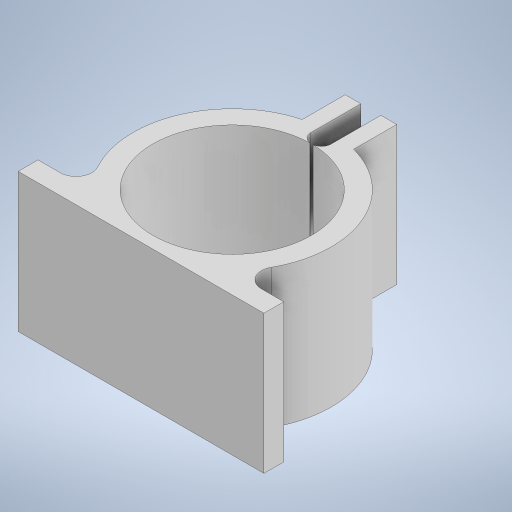
# Autodesk Inventor part: MotorClamp
Saved by Autodesk Inventor 2024 (Build 280153000, 153)
## iProperties
Created: 2023-08-28
Part Number: MotorClamp
Material: Generic
Document SubType Name: Modeling
Designer: KirikDK
Density: 1 g/cm^3
Appearance: Default
Author: KirikDK
Autodesk Inventor part; units mm, degrees
ref_plane "YZ Plane" through (0, 0, 0) normal (1, 0, 0) x (0, 1, 0)
ref_plane "XZ Plane" through (0, 0, 0) normal (0, 1, 0) x (-1, 0, 0)
ref_plane "XY Plane" through (0, 0, 0) normal (0, 0, 1) x (1, 0, 0)
sketch "Sketch1" plane through (0, 0, 0) normal (0, 1, 0) x (-1, 0, 0)
  circle A0 centre (0, 0) radius 50
  circle A1 centre (0, 0) radius 40
  line L0 (50, 0) -> (-50, 0)
  line L1 (-50, 0) -> (-50, 50)
  line L2 (-50, 50) -> (50, 50)
  line L3 (50, 50) -> (50, 0)
  line L4 (6, -46) -> (-6, -46)
  line L5 (-6, -46) -> (-6, -62)
  line L6 (-6, -62) -> (6, -62)
  line L7 (6, -62) -> (6, -46)
  line L8 (1, -64) -> (-1, -64)
  line L9 (-1, -64) -> (-1, -35)
  line L10 (-1, -35) -> (1, -35)
  line L11 (1, -35) -> (1, -64)
  point P0 (1, -39.9875)
  point P1 (1, -62)
  point P2 (6, -49.6387)
  point P3 (-6, -49.6387)
  point P4 (-1, -62)
  point P5 (-1, -39.9875)
  dimension "d0" = 100
  constraints: 24 end point, 6 parallel, 3 horizontal, 3 perpendicular, 2 coincident, 1 centre point, 3 other
extrude "Extrusion1" add sketch "Sketch1" along normal blind 70 contours L0 A1 A0 | A0 L7 L4 L11 A1 L0 | A0 L2 L3 | A0 L1 L2 | L7 L6 L11 A0 | A0 L11 L4 L7 | L0 A1 L9 L4 L5 A0 | L5 L4 L9 A0 | A0 L9 L6 L5
sketch "Sketch2" plane through (0, 70, 0) normal (0, 1, 0) x (1, 0, 0)
  circle A0 centre (0, 62) radius 3.05
  dimension "d9" = 6.1
  constraints: 1 centre point
  measures "d9" diameter of A0
extrude "Extrusion2" cut sketch "Sketch2" against normal blind 100
sketch "Sketch3" plane through (0, 70, 0) normal (0, 1, 0) x (1, 0, 0)
  line L0 (-3.05, 48) -> (-8, 48)
  line L1 (-8, 48) -> (-8, 62.2274)
  line L2 (-8, 62.2274) -> (-3.05, 62.2274)
  line L3 (-3.05, 62.2274) -> (-3.05, 48)
  line L4 (3.0501, 48) -> (8, 48)
  line L5 (8, 48) -> (8, 62.2274)
  line L6 (8, 62.2274) -> (3.0501, 62.2274)
  line L7 (3.0501, 62.2274) -> (3.0501, 48)
  constraints: 16 end point, 4 parallel, 2 horizontal, 2 perpendicular, 2 point on line
extrude "Extrusion3" add sketch "Sketch3" against normal up to surface (70 mm away)
sketch "Sketch4" plane through (0, 70, 0) normal (0, 1, 0) x (1, 0, 0)
  line L0 (8, 62.2274) -> (3.0501, 62.2274) construction
  line L1 (-3.05, 62.2274) -> (-8, 62.2274) construction
  arc A0 (-8, 49.3559) -> (-50, 0) centre (0, 0) ccw construction
  arc A1 (50, 0) -> (8, 49.3559) centre (0, 0) ccw construction
  line L2 (-8, 62.2274) -> (-20.0044, 45.8238)
  line L3 (8, 62.2274) -> (20.0044, 45.8238)
  line L4 (-20.0044, 45.8238) -> (-5.525, 45.8238)
  line L5 (-5.525, 45.8238) -> (-5.525, 62.2274)
  line L6 (-8, 62.2274) -> (-5.525, 62.2274)
  line L7 (20.0044, 45.8238) -> (5.5251, 45.8238)
  line L8 (5.5251, 45.8238) -> (5.5251, 62.2274)
  line L9 (5.5251, 62.2274) -> (8, 62.2274)
  constraints: 16 end point, 2 midpoint, 2 point on circle, 1 collinear, 1 horizontal, 1 perpendicular, 1 point on line
extrude "Extrusion4" add sketch "Sketch4" against normal blind 6
sketch "Sketch6" plane through (0, 70, 0) normal (0, 1, 0) x (1, 0, 0)
  line L0 (20, -36) -> (62, -36)
  line L1 (62, -36) -> (62, -50)
  line L2 (62, -50) -> (20, -50)
  line L3 (20, -50) -> (20, -36)
  line L4 (-22, -36) -> (-62, -36)
  line L5 (-62, -36) -> (-62, -50)
  line L6 (-62, -50) -> (-22, -50)
  line L7 (-22, -50) -> (-22, -36)
  point P0 (0, 0)
  constraints: 16 end point, 4 parallel, 2 horizontal, 2 perpendicular
extrude "Extrusion6" add sketch "Sketch6" against normal blind 70
sketch "Sketch7" plane through (0, 70, 0) normal (0, 1, 0) x (1, 0, 0)
  line L0 (-64, -52) -> (66, -52)
  line L1 (66, -52) -> (66, -46)
  line L2 (66, -46) -> (-64, -46)
  line L3 (-64, -46) -> (-64, -52)
  point P0 (0, 0)
  constraints: 8 end point, 2 parallel, 1 horizontal, 1 perpendicular
extrude "Extrusion7" cut sketch "Sketch7" against normal blind 70
sketch "Sketch8" plane through (8, 0, -62.2274) normal (0, 0, -1) x (-1, 0, 0)
  line L0 (0, 70) -> (4.9499, 70) projected
  line L1 (0, 70) -> (0, 64) projected
  line L2 (0, 64) -> (0, 0) projected
  line L3 (4.9499, 0) -> (0, 0) projected
  line L4 (4.9499, 70) -> (4.9499, 0) projected
  line L5 (16, 70) -> (16, 64) projected
  line L6 (11.05, 70) -> (16, 70) projected
  line L7 (11.05, 70) -> (11.05, 0) projected
  line L8 (16, 0) -> (11.05, 0) projected
  line L9 (16, 64) -> (16, 0) projected
  point P0 (8, 0)
extrude "Extrusion8" add sketch "Sketch8" along normal blind 10
sketch "Sketch9" plane through (0, 0, 0) normal (0, -1, 0) x (1, 0, 0)
  line L0 (5.0382, -76) -> (-5.0596, -76)
  line L1 (-5.0596, -76) -> (-5.0596, -32.6082)
  line L2 (-5.0596, -32.6082) -> (5.0382, -32.6082)
  line L3 (5.0382, -32.6082) -> (5.0382, -76)
  line L4 (-8, -62.2274) -> (-8, -72.2274) projected
  line L5 (-8, -72.2274) -> (-12, -72.2274)
  line L6 (-12, -72.2274) -> (-12, -46)
  line L7 (-12, -46) -> (-8, -46)
  line L8 (-8, -46) -> (-8, -72.2274)
  line L9 (8, -62.2274) -> (8, -72.2274) projected
  line L10 (8, -72.2274) -> (12, -72.2274)
  line L11 (12, -72.2274) -> (12, -47)
  line L12 (12, -47) -> (8, -47)
  line L13 (8, -47) -> (8, -72.2274)
  arc A0 (8, -49.3559) -> (50, 0) centre (0, 0) ccw projected
  circle A1 centre (0, 0) radius 50
  line L14 (-50, 36) -> (-62, 36) projected
  line L15 (60, 0) -> (-53, 0)
  line L16 (-53, 0) -> (-53, 36)
  line L17 (-53, 36) -> (60, 36)
  line L18 (60, 36) -> (60, 0)
  point P0 (-34.6987, 36)
  point P1 (-50, 0)
  point P2 (34.6987, 36)
  point P3 (50, 0)
  constraints: 32 end point, 8 parallel, 4 horizontal, 4 perpendicular, 1 coincident, 1 point on line, 3 other
extrude "Extrusion9" cut sketch "Sketch9" against normal blind 70 contours L0 L1 A1 L3 | A1 L1 L2 L3 | A1 L17 L18 L15 | L15 L16 L14 L17 A1
sketch "Sketch10" plane through (0, 0, 0) normal (0, -1, 0) x (1, 0, 0)
  point P0 (0, 0)
fillet "Fillet1" radius 8 2 edges at (34.6987, 35, 36) (-34.6987, 35, 36)
sketch "Sketch11" plane through (0, 0, 0) normal (0, -1, 0) x (1, 0, 0)
  line L0 (5.0382, -72.2274) -> (5.0382, -39.6814) projected
  line L1 (5.0382, -39.6814) -> (13, -39.6814)
  line L2 (13, -39.6814) -> (13, -72.2274)
  line L3 (13, -72.2274) -> (5.0382, -72.2274)
  line L4 (5.0382, -72.2274) -> (5.0382, -39.6814)
  line L5 (-5.0596, -72.2274) -> (-5.0596, -39.6787) projected
  line L6 (-5.0596, -72.2274) -> (-12.9756, -72.2274)
  line L7 (-12.9756, -72.2274) -> (-12.9756, -40)
  line L8 (-12.9756, -40) -> (-5.0596, -40)
  line L9 (-5.0596, -40) -> (-5.0596, -72.2274)
  point P0 (0, 0)
  point P1 (-5.0596, -40)
  constraints: 16 end point, 4 parallel, 2 horizontal, 2 perpendicular
extrude "Extrusion10" add sketch "Sketch11" against normal blind 70
sketch "Sketch12" plane through (0, 0, 0) normal (0, -1, 0) x (1, 0, 0)
  line L0 (13, -55.3951) -> (20.0044, -45.8238) projected
  line L1 (-12.9756, -55.4285) -> (-12.9756, -48.287) projected
  arc A0 (-20.0044, -45.8238) -> (-12.9756, -48.287) centre (0, 0) ccw projected
  line L2 (-20.0044, -45.8238) -> (-12.9756, -55.4285) projected
  line L3 (13, -48.2804) -> (13, -55.3951) projected
  line L4 (13, -55.3951) -> (20.0044, -45.8238) projected
  arc A1 (13, -48.2804) -> (20.0044, -45.8238) centre (0, 0) ccw projected
  line L5 (16, -74) -> (-16, -74)
  line L6 (-16, -74) -> (-16, -70)
  line L7 (-16, -70) -> (16, -70)
  line L8 (16, -70) -> (16, -74)
  constraints: 8 end point, 2 parallel, 1 horizontal, 1 perpendicular
extrude "Extrusion11" cut sketch "Sketch12" against normal blind 70
sketch "Sketch13" plane through (0, 0, 0) normal (0, -1, 0) x (1, 0, 0)
  circle A0 centre (0, -45) radius 5.0735
  circle A1 centre (0, 0) radius 40
  line L0 (5.0382, -70) -> (5.0382, -39.6814) projected
  line L1 (-5.0596, -39.6787) -> (-5.0596, -70) projected
  line L2 (5.0382, -52.0031) -> (-5.0596, -52.0031)
  line L3 (-5.0596, -52.0031) -> (-5.0596, -39.6787)
  line L4 (-5.0596, -39.6787) -> (5.0382, -39.6787)
  line L5 (5.0382, -39.6787) -> (5.0382, -52.0031)
  point P0 (5.0382, -44.4019)
  point P1 (0.8114, -39.9918)
  point P2 (-5.0596, -44.6244)
  point P3 (-0.8114, -39.9918)
  constraints: 8 end point, 2 centre point, 2 parallel, 1 coincident, 1 horizontal, 1 perpendicular, 1 point on line
extrude "Extrusion12" add sketch "Sketch13" against normal blind 70 contours A0 A1 L0 | A0 L1 A1
body "Solid1"
